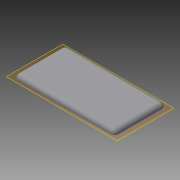
# Autodesk Inventor part: NanoCaseTop
Saved by Autodesk Inventor 2014 SP1 (Build 180222100, 222)
## iProperties
Created: 2017-05-21
Part Number: NanoCaseTop
Material: Generic
Document SubType Name: Modeling
Designer: danielsikar
Density: 1 g/cm^3
Appearance: Default
Author: danielsikar
Autodesk Inventor part; units mm, degrees
ref_plane "YZ Plane" through (0, 0, 0) normal (1, 0, 0) x (0, 1, 0)
ref_plane "XZ Plane" through (0, 0, 0) normal (0, 1, 0) x (-1, 0, 0)
ref_plane "Work Plane1" through (0, 0, 0) normal (0, 0, 1) x (1, 0, 0)
sketch "Sketch1" plane through (0, 0, 0) normal (0, 0, 1) x (1, 0, 0)
  line L0 (21.91, 12.18) -> (-21.91, 12.18) projected
  arc A0 (-23.91, -10.18) -> (-21.91, -12.18) centre (-21.91, -10.18) ccw projected
  line L1 (-21.91, -12.18) -> (21.91, -12.18) projected
  arc A1 (21.91, -12.18) -> (23.91, -10.18) centre (21.91, -10.18) ccw projected
  line L2 (23.91, -10.18) -> (23.91, -3.9) projected
  line L3 (23.91, -3.9) -> (22.39, -3.9) projected
  line L4 (22.39, -3.9) -> (22.39, -10.18) projected
  line L5 (22.39, -10.18) -> (-21.91, -10.18) projected
  line L6 (-21.91, -10.18) -> (-21.91, 10.18) projected
  line L7 (-21.91, 10.18) -> (22.39, 10.18) projected
  line L8 (22.39, 10.18) -> (22.39, 8.28) projected
  line L9 (22.39, 8.28) -> (23.91, 8.28) projected
  line L10 (23.91, 8.28) -> (23.91, 10.18) projected
  arc A2 (23.91, 10.18) -> (21.91, 12.18) centre (21.91, 10.18) ccw projected
  line L11 (21.91, 12.18) -> (-21.91, 12.18) projected
  arc A3 (-21.91, 12.18) -> (-23.91, 10.18) centre (-21.91, 10.18) ccw projected
  line L12 (-23.91, 10.18) -> (-23.91, -10.18) projected
  point P0 (0, 0)
extrude "Extrusion1" add sketch "Sketch1" along normal blind 2
sketch "Sketch2" plane through (22.39, 8.28, 0) normal (0, -1, 0) x (1, 0, 0)
  line L0 (0, 0) -> (1.52, 0) projected
  line L1 (1.52, 0) -> (1.52, 2) projected
  line L2 (0, 2) -> (1.52, 2) projected
  line L3 (0, 0) -> (0, 2) projected
  point P0 (-22.39, 0)
extrude "Extrusion2" add sketch "Sketch2" along normal up to next
sketch "Sketch4" plane through (-21.91, 10.18, 0) normal (0, -1, 0) x (1, 0, 0)
  line L0 (0, 0) -> (44.3, 0) projected
  line L1 (44.3, 0) -> (44.3, 2) projected
  line L2 (0, 2) -> (44.3, 2) projected
  line L3 (0, 0) -> (0, 2) projected
  point P0 (21.91, 0)
extrude "Extrusion3" add sketch "Sketch4" along normal up to next
fillet "Fillet1" radius 2 8 edges at (-23.3242, 11.5942, 2) (-23.91, 0, 2) (-23.3242, -11.5942, 2) (0, -12.18, 2) (23.3242, -11.5942, 2) (23.91, 0, 2) (23.3242, 11.5942, 2) (0, 12.18, 2)
ref_plane "Work Plane2" through (-20.91, -9.18, -4.3) normal (0, 0, 1) x (1, 0, 0)
sketch "Sketch3" plane through (0, 0, 0) normal (0, 0, 1) x (1, 0, 0)
  line L0 (-21.91, 10.18) -> (-19.41, 10.18)
  line L1 (-19.41, 7.68) -> (-19.41, 10.18)
  line L2 (-21.91, 7.68) -> (-19.41, 7.68)
  line L3 (-21.91, 7.68) -> (-21.91, 10.18)
  line L4 (19.89, 10.18) -> (22.39, 10.18)
  line L5 (19.89, 10.18) -> (19.89, 7.68)
  line L6 (19.89, 7.68) -> (22.39, 7.68)
  line L7 (22.39, 10.18) -> (22.39, 7.68)
  line L8 (-19.41, -10.18) -> (-21.91, -10.18)
  line L9 (-19.41, -10.18) -> (-19.41, -7.68)
  line L10 (-19.41, -7.68) -> (-21.91, -7.68)
  line L11 (-21.91, -10.18) -> (-21.91, -7.68)
  line L12 (22.39, -7.68) -> (22.39, -10.18)
  line L13 (22.39, -7.68) -> (19.89, -7.68)
  line L14 (19.89, -7.68) -> (19.89, -10.18)
  line L15 (22.39, -10.18) -> (19.89, -10.18)
  point P0 (0, 0)
extrude "Extrusion4" add sketch "Sketch3" against normal up to surface (4.3 mm away)
body "Solid1"
